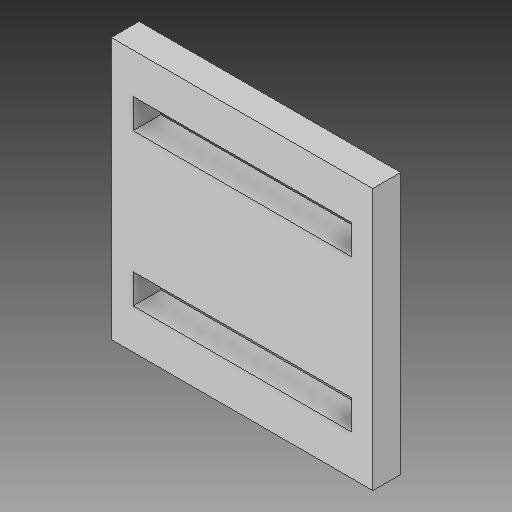
# Autodesk Inventor part: USBブリッジ基板1
Saved by Autodesk Inventor 2017 (Build 210142000, 142)
## iProperties
Created: 2016-08-22
Part Number: USBブリッジ基板1
Material: 一般
Document SubType Name: Modeling
Designer: NN
Density: 1 g/cm^3
Appearance: 既定
Mass: 0.292 g
Surface Area: 5.5188 cm^2
Volume: 0.292 cm^3
Author: NN
Autodesk Inventor part; units mm, degrees
ref_plane "YZ Plane" through (0, 0, 0) normal (1, 0, 0) x (0, 1, 0)
ref_plane "XZ Plane" through (0, 0, 0) normal (0, 1, 0) x (-1, 0, 0)
ref_plane "XY Plane" through (0, 0, 0) normal (0, 0, 1) x (1, 0, 0)
sketch "スケッチ1" plane through (0, 0, 0) normal (0, 0, 1) x (1, 0, 0)
  line L0 (0, 0) -> (15, 0)
  line L1 (15, 0) -> (15, 15)
  line L2 (15, 15) -> (0, 15)
  line L3 (0, 15) -> (0, 0)
  dimension "d0" = 15
  dimension "d1" = 15
  constraints: 8 end point, 2 parallel, 1 horizontal, 1 perpendicular
  measures "d0" distance of L0.start L0.end
  measures "d1" distance of L2.end L0.start
extrude "押し出し1" add sketch "スケッチ1" along normal blind 1.6
sketch "スケッチ2" plane through (0, 0, 1.6) normal (0, 0, 1) x (1, 0, 0)
  line L0 (1.25, 4) -> (13.75, 4)
  line L1 (13.75, 4) -> (13.75, 2.3)
  line L2 (13.75, 2.3) -> (1.25, 2.3)
  line L3 (1.25, 2.3) -> (1.25, 4)
  line L4 (0, 0) -> (15, 0) projected
  line L5 (15, 0) -> (15, 15) projected
  line L6 (15, 15) -> (0, 15) projected
  line L7 (0, 15) -> (0, 0) projected
  line L8 (0, 0) -> (15, 0) projected
  line L9 (0, 15) -> (0, 0) projected
  line L10 (0, 7.5) -> (2.3188, 7.5)
  line L11 (1.25, 11) -> (13.75, 11)
  line L12 (13.75, 11) -> (13.75, 12.7)
  line L13 (13.75, 12.7) -> (1.25, 12.7)
  line L14 (1.25, 12.7) -> (1.25, 11)
  line L15 (7.5, 2.3) -> (7.5, 0)
  point P0 (7.5, 13.5879)
  dimension "d4" = 12.5
  dimension "d5" = 1.7
  dimension "d6" = 7
  constraints: 20 end point, 4 symmetric about line, 3 midpoint, 2 horizontal, 2 parallel, 2 perpendicular
  measures "d4" distance of L12.end L13.end
  measures "d5" distance of L13.end L11.start
  measures "d6" distance between parallel lines of L0 L11
extrude "押し出し2" cut sketch "スケッチ2" against normal through all contours L0 L1 L2 L3 | L14 L13 L12 L11
